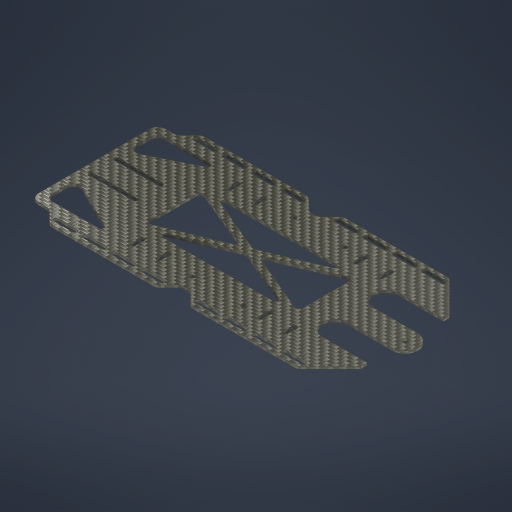
# Autodesk Inventor part: Tattu_Battery_Tray
Saved by Autodesk Inventor 2024 (Build 280153000, 153)
## iProperties
Created: 2023-06-19
Part Number: Tattu_Battery_Tray
Material: CFRP
Document SubType Name: Modeling
Designer: dzw04
Density: 1.43 g/cm^3
Appearance: Carbon Fiber 1
Author: dzw04
Autodesk Inventor part; units mm, degrees
ref_plane "YZ Plane" through (0, 0, 0) normal (1, 0, 0) x (0, 1, 0)
ref_plane "XZ Plane" through (0, 0, 0) normal (0, 1, 0) x (-1, 0, 0)
ref_plane "XY Plane" through (0, 0, 0) normal (0, 0, 1) x (1, 0, 0)
sketch "Sketch1" plane through (0, 0, 0) normal (0, 1, 0) x (-1, 0, 0)
  line L0 (-110, 36.5) -> (110, 36.5) construction
  line L1 (110, 36.5) -> (110, -36.5) construction
  line L2 (110, -36.5) -> (-110, -36.5) construction
  line L3 (-110, -36.5) -> (-110, 36.5) construction
  line L4 (-110, 36.5) -> (110, -36.5) construction
  line L5 (110, 36.5) -> (-110, -36.5) construction
  line L6 (-110, 29) -> (80, 29) construction
  line L7 (80, 29) -> (80, -29) construction
  line L8 (80, -29) -> (-110, -29) construction
  line L9 (-110, -29) -> (-110, 29) construction
  line L10 (-110, 29) -> (80, -29) construction
  line L11 (80, 29) -> (-110, -29) construction
  line L12 (-110, -29) -> (-110, -34) construction
  line L13 (-110, -34) -> (-60, -34) construction
  line L14 (-60, -34) -> (-50, -34) construction
  line L15 (-50, -34) -> (-70, -34) construction
  line L16 (-50, -34) -> (-50, -41.5) construction
  line L17 (-51.5, -34) -> (-51.5, -41.5)
  line L18 (-48.5, -41.5) -> (-48.5, -34)
  arc A0 (-48.5, -34) -> (-51.5, -34) centre (-50, -34) ccw
  arc A1 (-51.5, -41.5) -> (-48.5, -41.5) centre (-50, -41.5) ccw
  line L19 (-70, -34) -> (-70, -41.5) construction
  line L20 (-71.5, -34) -> (-71.5, -41.5)
  line L21 (-68.5, -41.5) -> (-68.5, -34)
  arc A2 (-68.5, -34) -> (-71.5, -34) centre (-70, -34) ccw
  arc A3 (-71.5, -41.5) -> (-68.5, -41.5) centre (-70, -41.5) ccw
  line L22 (122.5, 50) -> (-122.5, 50)
  line L23 (-122.5, 50) -> (-122.5, -50)
  line L24 (-122.5, -50) -> (122.5, -50)
  line L25 (122.5, -50) -> (122.5, 50)
  line L26 (122.5, 50) -> (-122.5, -50) construction
  line L27 (-122.5, 50) -> (122.5, -50) construction
  line L28 (122.5, 0) -> (-124.7912, 0) construction
  line L29 (-50, -34) -> (30, -34) construction
  line L30 (30, -34) -> (50, -34) construction
  line L31 (30, -34) -> (30, -41.5) construction
  line L32 (28.5, -34) -> (28.5, -41.5)
  line L33 (31.5, -41.5) -> (31.5, -34)
  arc A4 (31.5, -34) -> (28.5, -34) centre (30, -34) ccw
  arc A5 (28.5, -41.5) -> (31.5, -41.5) centre (30, -41.5) ccw
  line L34 (50, -34) -> (50, -41.5) construction
  line L35 (48.5, -34) -> (48.5, -41.5)
  line L36 (51.5, -41.5) -> (51.5, -34)
  arc A6 (51.5, -34) -> (48.5, -34) centre (50, -34) ccw
  arc A7 (48.5, -41.5) -> (51.5, -41.5) centre (50, -41.5) ccw
  line L37 (-110, 0) -> (80, 0) construction
  line L38 (80, 0) -> (80, -10) construction
  line L39 (80, 0) -> (80, 10) construction
  line L40 (80, -10) -> (115, -10) construction
  line L41 (80, -11.5) -> (115, -11.5)
  line L42 (115, -8.5) -> (80, -8.5)
  arc A8 (80, -8.5) -> (80, -11.5) centre (80, -10) ccw
  arc A9 (115, -11.5) -> (115, -8.5) centre (115, -10) ccw
  line L43 (80, 10) -> (115, 10) construction
  line L44 (80, 8.5) -> (115, 8.5)
  line L45 (115, 11.5) -> (80, 11.5)
  arc A10 (80, 11.5) -> (80, 8.5) centre (80, 10) ccw
  arc A11 (115, 8.5) -> (115, 11.5) centre (115, 10) ccw
  line L46 (-60, 34) -> (-50, 34) construction
  line L47 (-50, 34) -> (-70, 34) construction
  line L48 (-50, 34) -> (-50, 41.5) construction
  line L49 (-51.5, 34) -> (-51.5, 41.5)
  line L50 (-48.5, 41.5) -> (-48.5, 34)
  arc A12 (-51.5, 34) -> (-48.5, 34) centre (-50, 34) ccw
  arc A13 (-48.5, 41.5) -> (-51.5, 41.5) centre (-50, 41.5) ccw
  line L51 (-70, 34) -> (-70, 41.5) construction
  line L52 (-71.5, 34) -> (-71.5, 41.5)
  line L53 (-68.5, 41.5) -> (-68.5, 34)
  arc A14 (-71.5, 34) -> (-68.5, 34) centre (-70, 34) ccw
  arc A15 (-68.5, 41.5) -> (-71.5, 41.5) centre (-70, 41.5) ccw
  line L54 (-50, 34) -> (30, 34) construction
  line L55 (30, 34) -> (50, 34) construction
  line L56 (30, 34) -> (30, 41.5) construction
  line L57 (28.5, 34) -> (28.5, 41.5)
  line L58 (31.5, 41.5) -> (31.5, 34)
  arc A16 (28.5, 34) -> (31.5, 34) centre (30, 34) ccw
  arc A17 (31.5, 41.5) -> (28.5, 41.5) centre (30, 41.5) ccw
  line L59 (50, 34) -> (50, 41.5) construction
  line L60 (48.5, 34) -> (48.5, 41.5)
  line L61 (51.5, 41.5) -> (51.5, 34)
  arc A18 (48.5, 34) -> (51.5, 34) centre (50, 34) ccw
  arc A19 (51.5, 41.5) -> (48.5, 41.5) centre (50, 41.5) ccw
  circle A20 centre (-122.5, 0) radius 10
  point P0 (0, 0)
  point P1 (-15, 0)
  point P2 (-50, -37.75)
  point P3 (-70, -37.75)
  point P4 (30, -37.75)
  point P5 (50, -37.75)
  point P6 (97.5, -10)
  point P7 (97.5, 10)
  point P8 (-50, 37.75)
  point P9 (-70, 37.75)
  point P10 (30, 37.75)
  point P11 (50, 37.75)
  point P12 (-122.5, -10)
  point P13 (-122.5, 10)
  dimension "d0" = 220
  dimension "d1" = 73
  dimension "d2" = 190
  dimension "d3" = 58
  dimension "d4" = 5
  dimension "d5" = 50
  dimension "d6" = 10
  dimension "d7" = 20
  dimension "d8" = 7.5
  dimension "d9" = 3
  dimension "d10" = 7.5
  dimension "d11" = 3
  dimension "d12" = 245
  dimension "d13" = 100
  dimension "d16" = 80
  dimension "d17" = 20
  dimension "d18" = 7.5
  dimension "d19" = 3
  dimension "d20" = 7.5
  dimension "d21" = 3
  dimension "d22" = 10
  dimension "d23" = 10
  dimension "d24" = 35
  dimension "d25" = 3
  dimension "d26" = 35
  dimension "d27" = 3
  dimension "d52" = 20
  constraints: 144 end point, 40 point on circle, 29 symmetric about line, 24 tangent, 21 centre point, 17 midpoint, 14 parallel, 11 point on line, 8 perpendicular, 3 horizontal, 1 vertical, 8 other
  measures "d0" distance of L1.end L2.end
  measures "d1" distance of L0.end L1.end
  measures "d2" distance of L7.end L8.end
  measures "d3" distance of L6.end L7.end
  measures "d4" distance of L8.end L12.end
  measures "d5" distance of L12.end L13.end
  measures "d6" distance of L13.end L14.end
  measures "d7" distance of L14.end L15.end
  measures "d8" distance of L14.end L16.end
  measures "d9" diameter of A1
  measures "d10" distance of L15.end L19.end
  measures "d11" diameter of A3
  measures "d12" distance of L24.end L23.end
  measures "d13" distance of L23.end L22.end
  measures "d16" distance of L14.end L29.end
  measures "d17" distance of L29.end L30.end
  measures "d18" distance of L29.end L31.end
  measures "d19" diameter of A5
  measures "d20" distance of L30.end L34.end
  measures "d21" diameter of A7
  measures "d22" distance of L37.end L38.end
  measures "d23" distance of L37.end L39.end
  measures "d24" distance of L38.end L40.end
  measures "d25" diameter of A9
  measures "d26" distance of L39.end L43.end
  measures "d27" diameter of A11
  measures "d52" diameter of A20
extrude "Extrusion1" add sketch "Sketch1" along normal blind 1
sketch "Sketch2" plane through (0, 1, 0) normal (0, 1, 0) x (1, 0, 0)
  line L0 (0, 0) -> (55.5, 0) construction
  line L1 (55.5, 0) -> (55.5, -55) construction
  line L2 (55.5, -55) -> (51.5, -55) construction
  line L3 (51.5, -55) -> (36.5, -55) construction
  line L4 (51.5, -53.25) -> (36.5, -53.25)
  line L5 (36.5, -56.75) -> (51.5, -56.75)
  arc A0 (51.5, -56.75) -> (51.5, -53.25) centre (51.5, -55) ccw
  arc A1 (36.5, -53.25) -> (36.5, -56.75) centre (36.5, -55) ccw
  line L6 (36.5, -55) -> (28.5, -55) construction
  line L7 (28.5, -55) -> (13.5, -55) construction
  line L8 (28.5, -53.25) -> (13.5, -53.25)
  line L9 (13.5, -56.75) -> (28.5, -56.75)
  arc A2 (28.5, -56.75) -> (28.5, -53.25) centre (28.5, -55) ccw
  arc A3 (13.5, -53.25) -> (13.5, -56.75) centre (13.5, -55) ccw
  line L10 (0, 0) -> (0, -30) construction
  line L11 (55.5, -55) -> (59.5, -55) construction
  line L12 (59.5, -55) -> (74.5, -55) construction
  line L13 (59.5, -53.25) -> (74.5, -53.25)
  line L14 (74.5, -56.75) -> (59.5, -56.75)
  arc A4 (59.5, -53.25) -> (59.5, -56.75) centre (59.5, -55) ccw
  arc A5 (74.5, -56.75) -> (74.5, -53.25) centre (74.5, -55) ccw
  line L15 (74.5, -55) -> (82.5, -55) construction
  line L16 (82.5, -55) -> (97.5, -55) construction
  line L17 (82.5, -53.25) -> (97.5, -53.25)
  line L18 (97.5, -56.75) -> (82.5, -56.75)
  arc A6 (82.5, -53.25) -> (82.5, -56.75) centre (82.5, -55) ccw
  arc A7 (97.5, -56.75) -> (97.5, -53.25) centre (97.5, -55) ccw
  line L19 (-122.5, -50) -> (122.5, -50) projected
  line L20 (122.5, -50) -> (109.5711, -50)
  line L21 (107.5, -50) -> (107.5, -60) construction
  line L22 (107.5, -60) -> (97.5, -60) construction
  line L23 (98.9645, -58.5355) -> (106.0355, -51.4645)
  line L24 (95.4289, -60) -> (50.5, -60)
  arc A8 (95.4289, -60) -> (98.9645, -58.5355) centre (95.4289, -55) ccw
  arc A9 (109.5711, -50) -> (106.0355, -51.4645) centre (109.5711, -55) ccw
  line L25 (12.0355, -58.5355) -> (4.9645, -51.4645)
  line L26 (15.5711, -60) -> (50.5, -60)
  arc A10 (12.0355, -58.5355) -> (15.5711, -60) centre (15.5711, -55) ccw
  arc A11 (4.9645, -51.4645) -> (1.4289, -50) centre (1.4289, -55) ccw
  line L27 (-55.5, 0) -> (-55.5, -55) construction
  line L28 (-55.5, -55) -> (-51.5, -55) construction
  line L29 (-51.5, -55) -> (-36.5, -55) construction
  line L30 (-51.5, -53.25) -> (-36.5, -53.25)
  line L31 (-36.5, -56.75) -> (-51.5, -56.75)
  arc A12 (-51.5, -53.25) -> (-51.5, -56.75) centre (-51.5, -55) ccw
  arc A13 (-36.5, -56.75) -> (-36.5, -53.25) centre (-36.5, -55) ccw
  line L32 (-36.5, -55) -> (-28.5, -55) construction
  line L33 (-28.5, -55) -> (-13.5, -55) construction
  line L34 (-28.5, -53.25) -> (-13.5, -53.25)
  line L35 (-13.5, -56.75) -> (-28.5, -56.75)
  arc A14 (-28.5, -53.25) -> (-28.5, -56.75) centre (-28.5, -55) ccw
  arc A15 (-13.5, -56.75) -> (-13.5, -53.25) centre (-13.5, -55) ccw
  line L36 (-74.5, -56.75) -> (-59.5, -56.75)
  arc A16 (-59.5, -56.75) -> (-59.5, -53.25) centre (-59.5, -55) ccw
  arc A17 (-74.5, -53.25) -> (-74.5, -56.75) centre (-74.5, -55) ccw
  line L37 (-74.5, -55) -> (-82.5, -55) construction
  arc A18 (-82.5, -56.75) -> (-82.5, -53.25) centre (-82.5, -55) ccw
  line L38 (-97.5, -56.75) -> (-82.5, -56.75)
  arc A19 (-97.5, -53.25) -> (-97.5, -56.75) centre (-97.5, -55) ccw
  line L39 (-82.5, -55) -> (-97.5, -55) construction
  line L40 (-82.5, -53.25) -> (-97.5, -53.25)
  line L41 (-59.5, -55) -> (-74.5, -55) construction
  line L42 (-59.5, -53.25) -> (-74.5, -53.25)
  line L43 (-55.5, -55) -> (-59.5, -55) construction
  line L44 (122.5, -50) -> (-122.5, -50)
  line L45 (-122.5, -50) -> (-109.5711, -50)
  line L46 (-107.5, -50) -> (-107.5, -60) construction
  line L47 (-107.5, -60) -> (-97.5, -60) construction
  line L48 (-98.9645, -58.5355) -> (-106.0355, -51.4645)
  line L49 (-95.4289, -60) -> (-50.5, -60)
  arc A20 (-98.9645, -58.5355) -> (-95.4289, -60) centre (-95.4289, -55) ccw
  arc A21 (-106.0355, -51.4645) -> (-109.5711, -50) centre (-109.5711, -55) ccw
  line L50 (-15.5711, -60) -> (-50.5, -60)
  arc A22 (-15.5711, -60) -> (-12.0355, -58.5355) centre (-15.5711, -55) ccw
  line L51 (-12.0355, -58.5355) -> (-4.9645, -51.4645)
  arc A23 (-1.4289, -50) -> (-4.9645, -51.4645) centre (-1.4289, -55) ccw
  line L52 (55.5, 0) -> (55.5, 55) construction
  line L53 (55.5, 55) -> (51.5, 55) construction
  line L54 (51.5, 55) -> (36.5, 55) construction
  line L55 (51.5, 53.25) -> (36.5, 53.25)
  line L56 (36.5, 56.75) -> (51.5, 56.75)
  arc A24 (51.5, 53.25) -> (51.5, 56.75) centre (51.5, 55) ccw
  arc A25 (36.5, 56.75) -> (36.5, 53.25) centre (36.5, 55) ccw
  line L57 (36.5, 55) -> (28.5, 55) construction
  line L58 (28.5, 55) -> (13.5, 55) construction
  line L59 (28.5, 53.25) -> (13.5, 53.25)
  line L60 (13.5, 56.75) -> (28.5, 56.75)
  arc A26 (28.5, 53.25) -> (28.5, 56.75) centre (28.5, 55) ccw
  arc A27 (13.5, 56.75) -> (13.5, 53.25) centre (13.5, 55) ccw
  line L61 (74.5, 56.75) -> (59.5, 56.75)
  arc A28 (59.5, 56.75) -> (59.5, 53.25) centre (59.5, 55) ccw
  arc A29 (74.5, 53.25) -> (74.5, 56.75) centre (74.5, 55) ccw
  line L62 (74.5, 55) -> (82.5, 55) construction
  arc A30 (82.5, 56.75) -> (82.5, 53.25) centre (82.5, 55) ccw
  line L63 (97.5, 56.75) -> (82.5, 56.75)
  arc A31 (97.5, 53.25) -> (97.5, 56.75) centre (97.5, 55) ccw
  line L64 (82.5, 55) -> (97.5, 55) construction
  line L65 (82.5, 53.25) -> (97.5, 53.25)
  line L66 (59.5, 55) -> (74.5, 55) construction
  line L67 (59.5, 53.25) -> (74.5, 53.25)
  line L68 (55.5, 55) -> (59.5, 55) construction
  line L69 (-122.5, 50) -> (122.5, 50)
  line L70 (122.5, 50) -> (109.5711, 50)
  line L71 (107.5, 50) -> (107.5, 60) construction
  line L72 (107.5, 60) -> (97.5, 60) construction
  line L73 (98.9645, 58.5355) -> (106.0355, 51.4645)
  line L74 (95.4289, 60) -> (50.5, 60)
  arc A32 (98.9645, 58.5355) -> (95.4289, 60) centre (95.4289, 55) ccw
  arc A33 (106.0355, 51.4645) -> (109.5711, 50) centre (109.5711, 55) ccw
  line L75 (15.5711, 60) -> (50.5, 60)
  arc A34 (15.5711, 60) -> (12.0355, 58.5355) centre (15.5711, 55) ccw
  line L76 (12.0355, 58.5355) -> (4.9645, 51.4645)
  arc A35 (1.4289, 50) -> (4.9645, 51.4645) centre (1.4289, 55) ccw
  line L77 (-55.5, 55) -> (-51.5, 55) construction
  line L78 (-36.5, 55) -> (-28.5, 55) construction
  line L79 (122.5, 50) -> (-122.5, 50)
  line L80 (-15.5711, 60) -> (-50.5, 60)
  arc A36 (-36.5, 53.25) -> (-36.5, 56.75) centre (-36.5, 55) ccw
  line L81 (-51.5, 55) -> (-36.5, 55) construction
  line L82 (-36.5, 56.75) -> (-51.5, 56.75)
  arc A37 (-51.5, 56.75) -> (-51.5, 53.25) centre (-51.5, 55) ccw
  arc A38 (-59.5, 53.25) -> (-59.5, 56.75) centre (-59.5, 55) ccw
  line L83 (-51.5, 53.25) -> (-36.5, 53.25)
  arc A39 (-28.5, 56.75) -> (-28.5, 53.25) centre (-28.5, 55) ccw
  line L84 (-28.5, 53.25) -> (-13.5, 53.25)
  line L85 (-28.5, 55) -> (-13.5, 55) construction
  line L86 (-13.5, 56.75) -> (-28.5, 56.75)
  arc A40 (-13.5, 53.25) -> (-13.5, 56.75) centre (-13.5, 55) ccw
  arc A41 (-12.0355, 58.5355) -> (-15.5711, 60) centre (-15.5711, 55) ccw
  line L87 (-12.0355, 58.5355) -> (-4.9645, 51.4645)
  arc A42 (-4.9645, 51.4645) -> (-1.4289, 50) centre (-1.4289, 55) ccw
  line L88 (-55.5, 0) -> (-55.5, 55) construction
  line L89 (-59.5, 55) -> (-74.5, 55) construction
  arc A43 (-74.5, 56.75) -> (-74.5, 53.25) centre (-74.5, 55) ccw
  line L90 (-74.5, 55) -> (-82.5, 55) construction
  arc A44 (-82.5, 53.25) -> (-82.5, 56.75) centre (-82.5, 55) ccw
  line L91 (-82.5, 53.25) -> (-97.5, 53.25)
  line L92 (-82.5, 55) -> (-97.5, 55) construction
  line L93 (-97.5, 56.75) -> (-82.5, 56.75)
  arc A45 (-97.5, 56.75) -> (-97.5, 53.25) centre (-97.5, 55) ccw
  line L94 (-74.5, 56.75) -> (-59.5, 56.75)
  line L95 (-55.5, 55) -> (-59.5, 55) construction
  line L96 (-59.5, 53.25) -> (-74.5, 53.25)
  arc A46 (-95.4289, 60) -> (-98.9645, 58.5355) centre (-95.4289, 55) ccw
  line L97 (-98.9645, 58.5355) -> (-106.0355, 51.4645)
  line L98 (-107.5, 50) -> (-107.5, 60) construction
  line L99 (-107.5, 60) -> (-97.5, 60) construction
  arc A47 (-109.5711, 50) -> (-106.0355, 51.4645) centre (-109.5711, 55) ccw
  line L100 (-122.5, 50) -> (-109.5711, 50)
  line L101 (-95.4289, 60) -> (-50.5, 60)
  line L102 (122.5, 10) -> (122.5, 50) projected
  line L103 (122.5, 10) -> (87.5, 10)
  line L104 (122.5, -50) -> (122.5, -10) projected
  line L105 (122.5, -10) -> (87.5, -10)
  line L106 (87.5, 10) -> (87.5, 30) construction
  line L107 (87.5, -10) -> (87.5, -30) construction
  line L108 (87.5, 30) -> (122.5, 30)
  line L109 (87.5, -30) -> (122.5, -30)
  arc A48 (87.5, 30) -> (87.5, 10) centre (87.5, 20) ccw
  arc A49 (87.5, -10) -> (87.5, -30) centre (87.5, -20) ccw
  point P0 (44, -55)
  point P1 (21, -55)
  point P2 (67, -55)
  point P3 (90, -55)
  point P4 (-44, -55)
  point P5 (-21, -55)
  point P6 (-90, -55)
  point P7 (-67, -55)
  point P8 (44, 55)
  point P9 (21, 55)
  point P10 (90, 55)
  point P11 (67, 55)
  point P12 (-44, 55)
  point P13 (-21, 55)
  point P14 (-90, 55)
  point P15 (-67, 55)
  point P16 (1.4289, 50)
  point P17 (109.5711, 50)
  point P18 (-109.5711, 50)
  point P19 (-1.4289, 50)
  point P20 (-1.4289, -50)
  point P21 (-109.5711, -50)
  point P22 (109.5711, -50)
  point P23 (1.4289, -50)
  dimension "d28" = 55.5
  dimension "d29" = 55
  dimension "d30" = 4
  dimension "d31" = 15
  dimension "d32" = 3.5
  dimension "d33" = 8
  dimension "d34" = 15
  dimension "d35" = 3.5
  dimension "d36" = 30
  dimension "d37" = 15
  dimension "d38" = 10
  dimension "d39" = 10
  dimension "d40" = 5
  dimension "d53" = 35
  dimension "d54" = 35
  dimension "d55" = 20
  dimension "d56" = 20
  constraints: 246 end point, 162 symmetric about line, 100 point on circle, 50 centre point, 28 point on line, 12 tangent, 7 horizontal, 6 midpoint, 4 vertical, 2 parallel, 2 perpendicular, 1 equal radius, 42 other
  measures "d28" distance of L0.start L0.end
  measures "d29" distance of L0.end L1.end
  measures "d30" distance of L1.end L2.end
  measures "d31" distance of L2.end L3.end
  measures "d32" diameter of A1
  measures "d33" distance of L3.end L6.end
  measures "d34" distance of L6.end L7.end
  measures "d35" diameter of A3
  measures "d36" distance of L0.start L10.end
  measures "d37" distance of L19.end L21.start
  measures "d38" distance of L21.start L21.end
  measures "d39" distance of L21.end L22.end
  measures "d40" radius of A8
  measures "d53" distance of L102.start L103.end
  measures "d54" distance of L104.end L105.end
  measures "d55" distance of L103.end L106.end
  measures "d56" distance of L105.end L107.end
extrude "Extrusion2" add sketch "Sketch2" against normal blind 1 contours L19 A23 L51 A22 L50 L49 A20 L48 A21 | L19 A9 L23 A8 L24 L26 A10 L25 A11 | A47 L97 A46 L101 L80 A41 L87 A42 L69 | A35 L76 A34 L75 L74 A32 L73 A33 L69
sketch "Sketch3" plane through (0, 1, 0) normal (0, 1, 0) x (1, 0, 0)
  line L0 (98.9645, -58.5355) -> (106.0355, -51.4645) projected
  line L1 (106.0355, -51.4645) -> (137.8553, -19.6447)
  line L2 (106.0355, -51.4645) -> (151.0355, -51.4645) construction
  line L3 (106.0355, 51.4645) -> (137.8553, 19.6447)
  line L4 (106.0355, 51.4645) -> (151.0355, 51.4645) construction
  line L5 (106.0355, -51.4645) -> (127.5, -51.4645)
  line L6 (127.5, -51.4645) -> (127.5, -30)
  line L7 (127.5, -30) -> (106.0355, -30)
  line L8 (106.0355, -30) -> (106.0355, -51.4645)
  line L9 (106.0355, 51.4645) -> (127.5, 51.4645)
  line L10 (127.5, 51.4645) -> (127.5, 30)
  line L11 (127.5, 30) -> (106.0355, 30)
  line L12 (106.0355, 30) -> (106.0355, 51.4645)
  arc A0 (122.5, -10) -> (122.5, 10) centre (122.5, 0) ccw projected
  line L13 (122.5, 10) -> (87.5, 10)
  line L14 (87.5, 10) -> (87.5, 30) construction
  line L15 (87.5, 30) -> (122.5, 30)
  line L16 (122.5, 30) -> (122.5, 10)
  line L17 (122.5, -10) -> (87.5, -10)
  line L18 (87.5, -10) -> (87.5, -30) construction
  line L19 (87.5, -30) -> (122.5, -30)
  line L20 (122.5, -30) -> (122.5, -10)
  arc A1 (87.5, 30) -> (87.5, 10) centre (87.5, 20) ccw
  arc A2 (87.5, -10) -> (87.5, -30) centre (87.5, -20) ccw
  point P0 (0, 0)
  point P1 (122.5, 50)
  point P2 (106.0355, -30)
  point P3 (122.5, -30)
  point P4 (122.5, 30)
  point P5 (106.0355, 30)
  dimension "d43" = 45
  dimension "d44" = 45
  dimension "d45" = 45
  dimension "d46" = 45
  dimension "d57" = 35
  dimension "d58" = 20
  dimension "d59" = 35
  dimension "d60" = 20
  constraints: 40 end point, 8 parallel, 6 horizontal, 4 perpendicular, 4 point on circle, 2 centre point, 2 equal length, 2 midpoint, 2 point on line
  measures "d43" distance of L0.end L1.end
  measures "d44" angle of L2 L1
  measures "d45" distance of L3.start L3.end
  measures "d46" angle of L3 L4
  measures "d57" distance of L14.end L15.end
  measures "d58" distance of L13.end L14.end
  measures "d59" distance of L19.end L18.end
  measures "d60" distance of L18.end L17.end
extrude "Extrusion3" cut sketch "Sketch3" against normal blind 1 contours L1 L6 L5 | L19 A2 L17 L20 L7 | L9 L10 L3 | L11 L16 L13 A1 L15
fillet "Fillet1" radius 6 2 edges at (-122.5, 0.5, -50) (-122.5, 0.5, 50)
sketch "Sketch5" plane through (0, 1, 0) normal (0, 1, 0) x (1, 0, 0)
  line L0 (0, 0) -> (15, 0) construction
  line L1 (35, -40) -> (-5, -40) construction
  line L2 (-5, -40) -> (-5, 40) construction
  line L3 (-5, 40) -> (35, 40) construction
  line L4 (35, 40) -> (35, -40) construction
  line L5 (35, -40) -> (-5, 40) construction
  line L6 (-5, -40) -> (35, 40) construction
  circle A0 centre (35, -40) radius 1.75
  circle A1 centre (35, 40) radius 1.75
  circle A2 centre (-5, 40) radius 1.75
  circle A3 centre (-5, -40) radius 1.75
  dimension "d61" = 15
  dimension "d62" = 40
  dimension "d63" = 80
  dimension "d64" = 3.5
  dimension "d65" = 3.5
  dimension "d66" = 3.5
  dimension "d67" = 3.5
  constraints: 14 end point, 4 centre point, 4 coincident, 2 horizontal, 2 midpoint, 2 parallel, 1 perpendicular
  measures "d61" distance of L0.start L0.end
  measures "d62" distance of L2.end L3.end
  measures "d63" distance of L1.end L2.end
  measures "d64" diameter of A0
  measures "d65" diameter of A1
  measures "d66" diameter of A2
  measures "d67" diameter of A3
extrude "Extrusion4" cut sketch "Sketch5" against normal blind 1
sketch "Sketch6" plane through (0, 1, 0) normal (0, 1, 0) x (1, 0, 0)
  arc A0 (122.5, -10) -> (122.5, 10) centre (122.5, 0) ccw projected
  circle A1 centre (122.5, 0) radius 12.5
  circle A2 centre (122.5, 0) radius 2.35
  point P0 (0, 0)
  dimension "d70" = 25
  dimension "d71" = 4.7
  constraints: 2 centre point, 2 coincident
  measures "d70" diameter of A1
  measures "d71" diameter of A2
extrude "Extrusion5" cut sketch "Sketch6" against normal blind 1 contours A2
thicken "Thicken1" operation add thickness 1 both sides no extend neighbours no toward (0, -1, 0) faces at (8.5402, 0, -12.7879)
sketch "Sketch7" plane through (0, 1, 0) normal (0, 1, 0) x (1, 0, 0)
  line L0 (-43.5, -25) -> (43.5, -25)
  line L1 (60, -17.7917) -> (60, 17.7917)
  line L2 (43.5, 25) -> (-43.5, 25)
  line L3 (-60, 17.7917) -> (-60, -17.7917)
  line L4 (-60, -25) -> (60, 25) construction
  line L5 (60, -25) -> (-60, 25) construction
  line L6 (-55.8462, -20.5609) -> (-10.9308, -1.8462)
  line L7 (1.9231, 3.5096) -> (44.2692, 21.1538)
  line L8 (44.2692, -21.1538) -> (1.9231, -3.5096)
  line L9 (-10.9308, 1.8462) -> (-55.8462, 20.5609)
  line L10 (-44.2692, -21.1538) -> (-1.9231, -3.5096)
  line L11 (10.9308, 1.8462) -> (55.8462, 20.5609)
  line L12 (55.8462, -20.5609) -> (10.9308, -1.8462)
  line L13 (-1.9231, 3.5096) -> (-44.2692, 21.1538)
  arc A0 (-60, -17.7917) -> (-55.8462, -20.5609) centre (-57, -17.7917) ccw
  arc A1 (-55.8462, 20.5609) -> (-60, 17.7917) centre (-57, 17.7917) ccw
  arc A2 (60, 17.7917) -> (55.8462, 20.5609) centre (57, 17.7917) ccw
  arc A3 (55.8462, -20.5609) -> (60, -17.7917) centre (57, -17.7917) ccw
  arc A4 (43.5, -25) -> (44.2692, -21.1538) centre (43.5, -23) ccw
  arc A5 (44.2692, 21.1538) -> (43.5, 25) centre (43.5, 23) ccw
  arc A6 (-43.5, 25) -> (-44.2692, 21.1538) centre (-43.5, 23) ccw
  arc A7 (-44.2692, -21.1538) -> (-43.5, -25) centre (-43.5, -23) ccw
  arc A8 (10.9308, 1.8462) -> (10.9308, -1.8462) centre (11.7, 0) ccw
  arc A9 (-10.9308, -1.8462) -> (-10.9308, 1.8462) centre (-11.7, 0) ccw
  arc A10 (1.9231, -3.5096) -> (-1.9231, -3.5096) centre (0, -8.125) ccw
  arc A11 (-1.9231, 3.5096) -> (1.9231, 3.5096) centre (0, 8.125) ccw
  point P0 (0, 0)
  dimension "d76" = 120
  dimension "d77" = 50
  dimension "d82" = 3
  dimension "d83" = 2
  dimension "d84" = 5
  constraints: 28 end point, 24 point on circle, 24 tangent, 12 centre point, 10 parallel, 9 equal radius, 8 point on line, 2 midpoint, 1 horizontal, 1 perpendicular
  measures "d76" distance of L5.end L4.end
  measures "d77" distance of L4.end L5.start
  measures "d82" radius of A0
  measures "d83" radius of A4
  measures "d84" radius of A10
extrude "Extrusion6" cut sketch "Sketch7" against normal blind 3
sketch "Sketch8" plane through (0, 1, 0) normal (0, 1, 0) x (1, 0, 0)
  arc A0 (-116.5, 50) -> (-122.5, 44) centre (-116.5, 44) ccw projected
  line L0 (-111.5, 44) -> (-74.9721, 44)
  line L1 (-66.5, 44) -> (-66.5, 19) construction
  line L2 (-66.5, 19) -> (-116.5, 19) construction
  line L3 (-116.5, 27.0902) -> (-116.5, 39)
  arc A1 (-122.5, -44) -> (-116.5, -50) centre (-116.5, -44) ccw projected
  line L4 (-111.5, -44) -> (-74.9721, -44)
  line L5 (-66.5, -44) -> (-66.5, -19) construction
  line L6 (-66.5, -19) -> (-116.5, -19) construction
  line L7 (-116.5, -27.0902) -> (-116.5, -39)
  line L8 (-74.0777, -40.2111) -> (-109.2639, -22.618)
  line L9 (-109.2639, 22.618) -> (-74.0777, 40.2111)
  arc A2 (-116.5, -39) -> (-111.5, -44) centre (-111.5, -39) ccw
  arc A3 (-111.5, 44) -> (-116.5, 39) centre (-111.5, 39) ccw
  arc A4 (-109.2639, -22.618) -> (-116.5, -27.0902) centre (-111.5, -27.0902) ccw
  arc A5 (-116.5, 27.0902) -> (-109.2639, 22.618) centre (-111.5, 27.0902) ccw
  arc A6 (-74.9721, -44) -> (-74.0777, -40.2111) centre (-74.9721, -42) ccw
  arc A7 (-74.0777, 40.2111) -> (-74.9721, 44) centre (-74.9721, 42) ccw
  point P0 (0, 0)
  dimension "d87" = 50
  dimension "d88" = 25
  dimension "d89" = 50
  dimension "d90" = 25
  dimension "d91" = 5
  dimension "d92" = 5
  dimension "d93" = 2
  constraints: 20 end point, 12 point on circle, 12 point on line, 12 tangent, 6 centre point, 4 parallel, 3 equal radius, 2 horizontal, 2 perpendicular
  measures "d87" distance of L1.end L2.end
  measures "d88" distance of L1.start L1.end
  measures "d89" distance of L6.end L5.end
  measures "d90" distance of L5.end L5.start
  measures "d91" radius of A2
  measures "d92" radius of A4
  measures "d93" radius of A6
extrude "Extrusion7" cut sketch "Sketch8" against normal through all
body "Solid1"
